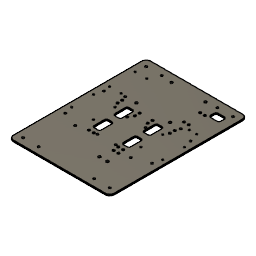
layer2_plate_v0_1 (Autodesk Fusion 360 design; units mm, degrees)
part number: 2026-05-30-13-28-22-122
Autodesk Fusion 360 part; units mm, degrees
box "长方体基本要素1" add length 285 width 145 height 3 placed x (0, 0, 1) y (1, 0, 0) z (0, 1, 0) at (0, 0, 0)
sketch "草图2" plane through (0, 3, 0) normal (0, 1, 0) x (-1, 0, 0)
  line L0 (0, 285) -> (-145, 285)
  line L1 (-145, 285) -> (-145, 0) construction
  line L2 (-145, 0) -> (0, 0)
  line L3 (0, 0) -> (0, 285) construction
  line L4 (0, 142.5) -> (-145, 142.5) construction
  line L5 (-72.5, 0) -> (-72.5, 285) construction
  line L6 (-30.4, 10) -> (-114.6, 10)
  line L7 (-114.6, 10) -> (-114.6, 97.5)
  line L8 (-114.6, 97.5) -> (-30.4, 97.5)
  line L9 (-30.4, 97.5) -> (-30.4, 10)
  line L10 (22.3, 32.5) -> (-7.7, 32.5)
  line L11 (-7.7, 32.5) -> (-7.7, 92.5)
  line L12 (-7.7, 92.5) -> (22.3, 92.5)
  line L13 (22.3, 92.5) -> (22.3, 32.5)
  line L14 (-137.6, 57.5) -> (-159.6, 57.5)
  line L15 (-159.6, 57.5) -> (-159.6, 87.5)
  line L16 (-159.6, 87.5) -> (-137.6, 87.5)
  line L17 (-137.6, 87.5) -> (-137.6, 57.5)
  line L18 (-50.8, 122.5) -> (-94.2, 122.5)
  line L19 (-94.2, 122.5) -> (-94.2, 189.43)
  line L20 (-94.2, 189.43) -> (-50.8, 189.43)
  line L21 (-50.8, 189.43) -> (-50.8, 122.5)
  line L22 (32.3, 0) -> (-177.3, 0)
  line L23 (32.3, 285) -> (-177.3, 285)
  line L24 (32.3, 0) -> (32.3, 285)
  line L25 (-177.3, 0) -> (-177.3, 285)
  line L26 (24.3, 117.5) -> (-25.7, 117.5)
  line L27 (-25.7, 167.5) -> (24.3, 167.5)
  line L28 (24.3, 167.5) -> (24.3, 117.5)
  line L29 (24.3, 142.5) -> (-24.8585, 142.5) construction
  line L30 (-25.7, 125) -> (-33.7, 125)
  line L31 (-33.7, 125) -> (-33.7, 160)
  line L32 (-33.7, 160) -> (-25.7, 160)
  line L33 (-25.7, 117.5) -> (-25.7, 125)
  line L34 (-25.7, 160) -> (-25.7, 167.5)
  line L35 (-169.3, 167.5) -> (-169.3, 117.5)
  line L36 (-169.3, 117.5) -> (-119.3, 117.5)
  line L37 (-119.3, 167.5) -> (-169.3, 167.5)
  line L38 (-119.3, 160) -> (-119.3, 167.5)
  line L39 (-111.3, 160) -> (-119.3, 160)
  line L40 (-111.3, 125) -> (-111.3, 160)
  line L41 (-119.3, 125) -> (-111.3, 125)
  line L42 (-119.3, 117.5) -> (-119.3, 125)
  line L43 (-38.25, 107) -> (-46.25, 107)
  line L44 (-49.25, 110) -> (-49.25, 132)
  line L45 (-46.25, 135) -> (-38.25, 135)
  line L46 (-35.25, 132) -> (-35.25, 110)
  arc A0 (-38.25, 107) -> (-35.25, 110) centre (-38.25, 110) ccw
  arc A1 (-49.25, 110) -> (-46.25, 107) centre (-46.25, 110) ccw
  arc A2 (-46.25, 135) -> (-49.25, 132) centre (-46.25, 132) ccw
  arc A3 (-35.25, 132) -> (-38.25, 135) centre (-38.25, 132) ccw
  line L47 (-33.7, 125) -> (-35.25, 125) construction
  line L48 (-50.8, 122.5) -> (-49.25, 122.5) construction
  line L49 (-35.25, 153) -> (-35.25, 175)
  arc A4 (-35.25, 175) -> (-38.25, 178) centre (-38.25, 175) ccw
  line L50 (-38.25, 178) -> (-46.25, 178)
  arc A5 (-46.25, 178) -> (-49.25, 175) centre (-46.25, 175) ccw
  line L51 (-49.25, 175) -> (-49.25, 153)
  arc A6 (-49.25, 153) -> (-46.25, 150) centre (-46.25, 153) ccw
  line L52 (-46.25, 150) -> (-38.25, 150)
  arc A7 (-38.25, 150) -> (-35.25, 153) centre (-38.25, 153) ccw
  line L53 (-106.75, 178) -> (-98.75, 178)
  line L54 (-106.75, 107) -> (-98.75, 107)
  arc A8 (-95.75, 132) -> (-98.75, 135) centre (-98.75, 132) ccw
  arc A9 (-98.75, 107) -> (-95.75, 110) centre (-98.75, 110) ccw
  arc A10 (-98.75, 150) -> (-95.75, 153) centre (-98.75, 153) ccw
  line L55 (-98.75, 150) -> (-106.75, 150)
  arc A11 (-109.75, 153) -> (-106.75, 150) centre (-106.75, 153) ccw
  line L56 (-109.75, 132) -> (-109.75, 110)
  arc A12 (-106.75, 135) -> (-109.75, 132) centre (-106.75, 132) ccw
  arc A13 (-95.75, 175) -> (-98.75, 178) centre (-98.75, 175) ccw
  line L57 (-98.75, 135) -> (-106.75, 135)
  arc A14 (-106.75, 178) -> (-109.75, 175) centre (-106.75, 175) ccw
  arc A15 (-109.75, 110) -> (-106.75, 107) centre (-106.75, 110) ccw
  line L58 (-95.75, 110) -> (-95.75, 132)
  line L59 (-95.75, 175) -> (-95.75, 153)
  line L60 (-109.75, 153) -> (-109.75, 175)
  line L61 (-92.5, 213.47) -> (-116.12, 213.47)
  line L62 (-116.12, 213.47) -> (-116.12, 245)
  line L63 (-116.12, 245) -> (-92.5, 245)
  line L64 (-92.5, 245) -> (-92.5, 213.47)
  line L65 (-140.3, 25) -> (-154.3, 25)
  line L66 (-157.3, 28) -> (-157.3, 36)
  line L67 (-154.3, 39) -> (-140.3, 39)
  line L68 (-137.3, 36) -> (-137.3, 28)
  circle A16 centre (-130, 15) radius 2.15
  circle A17 centre (-15, 15) radius 2.15
  circle A18 centre (-130, 270) radius 2.15
  circle A19 centre (-15, 270) radius 2.15
  arc A20 (-140.3, 25) -> (-137.3, 28) centre (-140.3, 28) ccw
  arc A21 (-137.3, 36) -> (-140.3, 39) centre (-140.3, 36) ccw
  arc A22 (-154.3, 39) -> (-157.3, 36) centre (-154.3, 36) ccw
  arc A23 (-157.3, 28) -> (-154.3, 25) centre (-154.3, 28) ccw
  circle A24 centre (-15, 90.825) radius 2.15
  circle A25 centre (-130, 90.825) radius 2.15
  circle A26 centre (-15, 194.175) radius 2.15
  circle A27 centre (-130, 194.175) radius 2.15
  circle A28 centre (17.3, 270) radius 2.15
  circle A29 centre (-162.3, 270) radius 2.15
  circle A30 centre (17.3, 15) radius 2.15
  circle A31 centre (-162.3, 15) radius 2.15
  circle A32 centre (17.3, 102.5) radius 2.15
  circle A33 centre (-162.3, 102.5) radius 2.15
  circle A34 centre (17.3, 182.5) radius 2.15
  circle A35 centre (-162.3, 182.5) radius 2.15
  circle A36 centre (19.3, 36) radius 1.75
  line L69 (22.3, 62.5) -> (-7.7, 62.5) construction
  line L70 (7.3, 32.5) -> (7.3, 92.5) construction
  circle A37 centre (-4.7, 36) radius 1.75
  circle A38 centre (19.3, 89) radius 1.75
  circle A39 centre (-4.7, 89) radius 1.75
  circle A40 centre (-141.1, 84) radius 1.65
  line L71 (-148.6, 57.5) -> (-148.6, 87.5) construction
  circle A41 centre (-156.1, 84) radius 1.65
  circle A42 centre (-96, 225.17) radius 2.65
  line L72 (-104.31, 213.47) -> (-104.31, 245) construction
  circle A43 centre (-112.62, 225.17) radius 2.65
  line L73 (-30.4, 53.75) -> (-114.6, 53.75) construction
  circle A44 centre (-37.6, 90.3) radius 2.5
  circle A45 centre (-107.4, 90.3) radius 2.5
  circle A46 centre (-37.6, 17.2) radius 2.5
  circle A47 centre (-107.4, 17.2) radius 2.5
  circle A48 centre (21.8, 120) radius 1.75
  line L74 (-0.7, 117.5) -> (-0.7, 167.5) construction
  line L75 (-0.7, 167.5) -> (-0.7, 117.5) construction
  circle A49 centre (21.8, 165) radius 1.75
  circle A50 centre (-23.2, 120) radius 1.75
  circle A51 centre (-23.2, 165) radius 1.75
  circle A52 centre (-166.8, 120) radius 1.75
  circle A53 centre (-121.8, 120) radius 1.75
  circle A54 centre (-166.8, 165) radius 1.75
  circle A55 centre (-121.8, 165) radius 1.75
  line L76 (-50.8, 155.965) -> (-94.2, 155.965) construction
  circle A56 centre (-53.6, 186.765) radius 2.15
  circle A57 centre (-91.4, 186.765) radius 2.15
  circle A58 centre (-53.6, 125.165) radius 2.15
  circle A59 centre (-91.4, 125.165) radius 2.15
  circle A60 centre (-131.1, 75.2117) radius 1.75
  circle A61 centre (-121.1, 75.2117) radius 1.75
  line L77 (-42.25, 150) -> (-42.25, 178) construction
  circle A62 centre (-37.25, 188) radius 1.75
  circle A63 centre (-107.75, 188) radius 1.75
  line L78 (-54.79, 110) -> (-91.4013, 110) construction
  circle A64 centre (-59.25, 105) radius 1.75
  circle A65 centre (-85.75, 105) radius 1.75
  circle A66 centre (-18.036, 100) radius 1.75
  line L79 (-114.6, 61.3197) -> (-137.6, 61.3197) construction
  line L80 (-126.1, 61.3197) -> (-126.1, 45.2779) construction
  circle A67 centre (-131.1, 41.8248) radius 1.75
  circle A68 centre (-121.1, 41.8248) radius 1.75
  circle A69 centre (-59.25, 115) radius 1.75
  circle A70 centre (-85.75, 115) radius 1.75
  circle A71 centre (-18.286, 110) radius 1.75
  circle A72 centre (-126.964, 100) radius 1.75
  circle A73 centre (-126.714, 110) radius 1.75
  circle A74 centre (-99.31, 199.046) radius 1.75
  circle A75 centre (-109.31, 199.046) radius 1.75
  circle A76 centre (-47.25, 188) radius 1.75
  circle A77 centre (-97.75, 188) radius 1.75
  point P0 (-109.75, 125)
  point P1 (-95.75, 122.5)
  point P2 (-137.3, 25)
  point P3 (-157.3, 25)
  point P4 (-137.3, 39)
  point P5 (-121.1, 75.2117)
  point P6 (-131.1, 75.2117)
  point P7 (-72.5, 97.5)
  point P8 (-72.5, 122.5)
  point P9 (-18.036, 100)
  point P10 (-131.1, 41.8248)
  point P11 (-121.1, 41.8248)
  dimension "d12" = 43.4
  dimension "d13" = 66.93
  dimension "d16" = 84.2
  dimension "d17" = 87.5
  dimension "d20" = 10
  dimension "d21" = 30
  dimension "d22" = 60
  dimension "d23" = 209.6
  dimension "d24" = 50
  dimension "d25" = 50
  dimension "d26" = 8
  dimension "d27" = 35
  dimension "d31" = 14
  dimension "d32" = 3
  dimension "d35" = 28
  dimension "d36" = 15
  dimension "d37" = 8
  dimension "d38" = 25
  dimension "d39" = 10
  dimension "d40" = 22
  dimension "d41" = 30
  dimension "d42" = 30
  dimension "d43" = 23
  dimension "d46" = 23.62
  dimension "d47" = 31.53
  dimension "d48" = 20
  dimension "d49" = 40
  dimension "d70" = 20
  dimension "d71" = 14
  dimension "d72" = 25
  dimension "d73" = 20
  dimension "d74" = 4.3
  dimension "d75" = 15
  dimension "d76" = 15
  dimension "d77" = 3
  dimension "d78" = 3
  dimension "d79" = 3
  dimension "d80" = 3
  dimension "d89" = 4.3
  dimension "d90" = 90.825
  dimension "d91" = 15
  dimension "d96" = 4.3
  dimension "d97" = 15
  dimension "d98" = 15
  dimension "d99" = 4.3
  dimension "d100" = 15
  dimension "d101" = 10
  dimension "d104" = 3.5
  dimension "d105" = 53
  dimension "d106" = 24
  dimension "d107" = 3.3
  dimension "d108" = 15
  dimension "d109" = 3.5
  dimension "d110" = 5.3
  dimension "d111" = 3.5
  dimension "d112" = 11.7
  dimension "d113" = 5
  dimension "d114" = 73.1
  dimension "d115" = 69.8
  dimension "d116" = 3.5
  dimension "d117" = 45
  dimension "d118" = 45
  dimension "d119" = 4.3
  dimension "d120" = 37.8
  dimension "d121" = 61.6
  dimension "d122" = 25
  dimension "d127" = 3.5
  dimension "d128" = 3.5
  dimension "d129" = 3.5
  dimension "d130" = 10
  dimension "d131" = 3.5
  dimension "d132" = 10
  dimension "d134" = 3.5
  dimension "d135" = 10
  dimension "d136" = 3.5
  dimension "d137" = 3.5
  dimension "d138" = 10
  dimension "d139" = 10
  dimension "d140" = 3.5
  dimension "d141" = 10
  dimension "d142" = 7.5
  dimension "d143" = 3.5
  dimension "d144" = 10
  dimension "d145" = 10
  constraint midpoint L3 L4.start
  constraint midpoint L1 L4.end
  constraint midpoint L2 L5.start
  constraint midpoint L0 L5.end
  constraint horizontal L6
  constraint vertical L7
  constraint horizontal L8
  constraint vertical L9
  constraint horizontal L10
  constraint vertical L11
  constraint horizontal L12
  constraint vertical L13
  constraint horizontal L14
  constraint vertical L15
  constraint horizontal L16
  constraint vertical L17
  constraint horizontal L18
  constraint vertical L19
  constraint horizontal L20
  constraint vertical L21
  constraint symmetric L5 L7 L9
  constraint parallel L6 L22
  constraint symmetric L5 L22.start L22.end
  constraint coincident L5.start L22
  constraint symmetric L4 L22.start L23.start
  constraint symmetric L4 L22.end L23.end
  constraint horizontal L26
  constraint vertical L33
  constraint horizontal L27
  constraint vertical L28
  constraint midpoint L28 L29.start
  constraint perpendicular L30 L33
  constraint perpendicular L4 L31
  constraint perpendicular L32 L34
  constraint symmetric L29 L30 L32
  constraint symmetric L4 L26 L27
  constraint collinear L33 L34
  constraint symmetric L5 L26.start L35.end
  constraint symmetric L5 L26.end L36.end
  constraint symmetric L5 L27.start L37.start
  constraint symmetric L5 L27.end L35.start
  constraint symmetric L5 L30.start L41.start
  constraint symmetric L5 L30.end L40.start
  constraint symmetric L5 L31.end L39.start
  constraint symmetric L5 L32.end L38.start
  constraint horizontal L43
  constraint vertical L44
  constraint horizontal L45
  constraint vertical L46
  constraint tangent L46 A0
  constraint tangent L43 A0
  constraint tangent L43 A1
  constraint tangent L44 A1
  constraint tangent L44 A2
  constraint tangent L45 A2
  constraint tangent L45 A3
  constraint tangent L46 A3
  constraint coincident L46 L47.end
  constraint perpendicular L46 L47
  constraint coincident L44 L48.end
  constraint perpendicular L44 L48
  constraint equal L47 L48
  constraint symmetric L5 L19 L21
  constraint symmetric L4 L46.end L49.end
  constraint symmetric L4 L43.start A4.end
  constraint symmetric L4 A0 A4
  constraint symmetric L4 L43.end L50.end
  constraint symmetric L4 L44.start A5.end
  constraint symmetric L4 A1 A5
  constraint symmetric L4 L44.end L51.end
  constraint symmetric L4 L45.start A6.end
  constraint symmetric L4 A2 A6
  constraint symmetric L4 L45.end L52.end
  constraint symmetric L4 L46.start L49.start
  constraint symmetric L4 A3 A7
  constraint symmetric L5 L46.end L56.end
  constraint symmetric L5 L43.start L54.start
  constraint symmetric L5 A0 A15
  constraint symmetric L5 L43.end L54.end
  constraint symmetric L5 L44.start A9.end
  constraint symmetric L5 A1 A9
  constraint symmetric L5 L44.end A8.start
  constraint symmetric L5 L45.start A8.end
  constraint symmetric L5 A2 A8
  constraint symmetric L5 L45.end A12.start
  constraint symmetric L5 L46.start L56.start
  constraint symmetric L5 A3 A12
  constraint symmetric L5 L47.end P0
  constraint symmetric L5 L48.end P1
  constraint symmetric L5 L49.start A11.start
  constraint symmetric L5 L49.end A14.end
  constraint symmetric L5 A4.end L53.start
  constraint symmetric L5 A4 A14
  constraint symmetric L5 L50.end L53.end
  constraint symmetric L5 A5.end A13.start
  constraint symmetric L5 A5 A13
  constraint symmetric L5 L51.end A10.end
  constraint symmetric L5 A6.end A10.start
  constraint symmetric L5 A6 A10
  constraint symmetric L5 L52.end L55.end
  constraint symmetric L5 A7 A11
  constraint equal A0 A1
  constraint equal A1 A3
  constraint equal A1 A2
  constraint horizontal L61
  constraint vertical L62
  constraint horizontal L63
  constraint vertical L64
  constraint horizontal L65
  constraint vertical L66
  constraint horizontal L67
  constraint vertical L68
  constraint symmetric L5 A16 A17
  constraint symmetric L4 A16 A18
  constraint symmetric L4 A17 A19
  constraint coincident P2 L68
  constraint coincident P2 L65
  constraint tangent L68 A20
  constraint tangent L65 A20
  constraint coincident P4 L67
  constraint coincident P4 L68
  constraint tangent L67 A21
  constraint tangent L68 A21
  constraint tangent L67 A22
  constraint tangent L66 A22
  constraint coincident P3 L65
  constraint coincident P3 L66
  constraint tangent L65 A23
  constraint tangent L66 A23
  constraint symmetric L5 A24 A25
  constraint symmetric L4 A24 A26
  constraint symmetric L4 A25 A27
  constraint symmetric L5 A28 A29
  constraint symmetric L4 A28 A30
  constraint symmetric L4 A29 A31
  constraint symmetric L5 A32 A33
  constraint symmetric L4 A32 A34
  constraint symmetric L4 A33 A35
  constraint midpoint L13 L69.start
  constraint midpoint L11 L69.end
  constraint midpoint L10 L70.start
  constraint midpoint L12 L70.end
  constraint symmetric A36 L70 A37
  constraint symmetric A36 L69 A38
  constraint symmetric L69 A37 A39
  constraint midpoint L14 L71.start
  constraint midpoint L16 L71.end
  constraint symmetric A40 L71 A41
  constraint midpoint L61 L72.start
  constraint midpoint L63 L72.end
  constraint symmetric A42 L72 A43
  constraint midpoint L9 L73.start
  constraint midpoint L7 L73.end
  constraint symmetric L5 A44 A45
  constraint symmetric L73 A44 A46
  constraint symmetric L73 A45 A47
  constraint midpoint L26 L74.start
  constraint midpoint L27 L74.end
  constraint symmetric L29 A48 A49
  constraint symmetric L29 L74.start L74.end
  constraint symmetric L29 L74.end L74.start
  constraint symmetric A48 L74 A50
  constraint symmetric L74 A49 A51
  constraint symmetric L5 A48 A52
  constraint symmetric L5 A49 A54
  constraint symmetric L5 A50 A53
  constraint symmetric L5 A51 A55
  constraint midpoint L21 L76.start
  constraint midpoint L19 L76.end
  constraint symmetric L5 A56 A57
  constraint symmetric L76 A56 A58
  constraint symmetric L76 A57 A59
  constraint coincident P6 A60.centre
  constraint coincident P5 A61.centre
  constraint midpoint L52 L77.start
  constraint midpoint L50 L77.end
  constraint symmetric L5 A62 A63
  constraint perpendicular L44 L78
  constraint midpoint L8 P7
  constraint midpoint L18 P8
  constraint symmetric L78 P7 P8
  constraint symmetric L5 A64 A65
  constraint coincident P9 A66.centre
  constraint coincident L7 L79.start
  constraint coincident L17 L79.end
  constraint perpendicular L17 L79
  constraint midpoint L79 L80.start
  constraint perpendicular L79 L80
  constraint symmetric P6 P5 L80
  constraint coincident P10 A67.centre
  constraint coincident P11 A68.centre
  constraint symmetric L80 P11 P10
  constraint symmetric L78 A64 A69
  constraint symmetric L78 A65 A70
  constraint symmetric L5 A66 A72
  constraint symmetric L5 A71 A73
  constraint symmetric L72 A74 A75
  constraint symmetric L77 A62 A76
  constraint symmetric L5 A76 A77
  measures "d12" distance of L19.end L20.end
  measures "d13" distance of L18.end L19.end
  measures "d16" distance of L7.end L8.end
  measures "d17" distance of L6.end L7.end
  measures "d20" distance of L2 L6
  measures "d21" distance of L11.end L12.end
  measures "d22" distance of L10.start L12.end
  measures "d23" distance of L22.start L22.end
  measures "d24" distance of L26.start L26.end
  measures "d25" distance of L26.start L27.end
  measures "d26" distance of L30.start L30.end
  measures "d27" distance of L30.end L31.end
  measures "d31" distance of L44 L46
  measures "d32" radius of A1
  measures "d35" distance of L43 L45
  measures "d36" distance of L45 L52
  measures "d37" distance of L24 L28
  measures "d38" distance of L12 L26
  measures "d39" distance of L13 L24
  measures "d40" distance of L14.start L14.end
  measures "d41" distance of L14.end L15.end
  measures "d42" distance of L16 L36
  measures "d43" distance of L7 L17
  measures "d46" distance of L62.end L63.end
  measures "d47" distance of L61.start L63.end
  measures "d48" distance of L5 L64
  measures "d49" distance of L23 L63
  measures "d70" distance of P2 P3
  measures "d71" distance of P2 P4
  measures "d72" distance of L22 P2
  measures "d73" distance of L25 L66
  measures "d74" diameter of A16
  measures "d75" distance of L22 A16.centre
  measures "d76" distance of L1 A16.centre
  measures "d77" radius of A20
  measures "d78" radius of A21
  measures "d79" radius of A22
  measures "d80" radius of A23
  measures "d89" diameter of A24
  measures "d90" distance of L22 A24.centre
  measures "d91" distance of L3 A24.centre
  measures "d96" diameter of A28
  measures "d97" distance of L24 A28.centre
  measures "d98" distance of L23 A28.centre
  measures "d99" diameter of A32
  measures "d100" distance of L24 A32.centre
  measures "d101" distance of L12 A32.centre
  measures "d104" diameter of A36
  measures "d105" distance of A36.centre A38.centre
  measures "d106" distance of A36.centre A37.centre
  measures "d107" diameter of A40
  measures "d108" distance of A40.centre A41.centre
  measures "d109" distance of L16 A40.centre
  measures "d110" diameter of A42
  measures "d111" distance of L64 A42.centre
  measures "d112" distance of L61 A42.centre
  measures "d113" diameter of A44
  measures "d114" distance of A44.centre A46.centre
  measures "d115" distance of A46.centre A47.centre
  measures "d116" diameter of A48
  measures "d117" distance of A48.centre A50.centre
  measures "d118" distance of A48.centre A49.centre
  measures "d119" diameter of A56
  measures "d120" distance of A56.centre A57.centre
  measures "d121" distance of A56.centre A58.centre
  measures "d122" distance of L8 L18
  measures "d127" diameter of A60
  measures "d128" diameter of A61
  measures "d129" diameter of A62
  measures "d130" distance of L50 A62.centre
  measures "d131" diameter of A64
  measures "d132" distance of L44 A64.centre
  measures "d134" diameter of A66
  measures "d135" distance of P5 P6
  measures "d136" diameter of A67
  measures "d137" diameter of A68
  measures "d138" distance of P10 P11
  measures "d139" distance of A64.centre A69.centre
  measures "d140" diameter of A71
  measures "d141" vertical distance of P9 A71.centre
  measures "d142" distance of L12 P9
  measures "d143" diameter of A74
  measures "d144" distance of A74.centre A75.centre
  measures "d145" distance of A62.centre A76.centre
extrude "拉伸3" add sketch "草图2" against normal blind 3 contours L0 L2 L22 L23 L24 L25 | L6 L7 L8 L9 | L10 L11 L12 L13 | L14 L15 L16 L17 | L18 L19 L20 L21 | L26 L27 L28 L30 L31 L32 L33 L34 | L35 L36 L37 L38 L39 L40 L41 L42 | L43 L44 L45 L46 A0 A1 A2 A3 | L49 A4 L50 A5 L51 A6 L52 A7 | L53 A10 L55 A11 A13 A14 L59 L60 | L54 A8 A9 L56 A12 L57 A15 L58 | L61 L62 L63 L64 | L65 L66 L67 L68 A20 A21 A22 A23 | A16 | A17 | A18 | A19 | A24 | A25 | A26 | A27 | A28 | A29 | A30 | A31 | A32 | A33 | A34 | A35 | A36 | A37 | A38 | A39 | A40 | A41 | A42 | A43 | A44 | A45 | A46 | A47 | A48 | A49 | A50 | A51 | A52 | A53 | A54 | A55 | A56 | A57 | A58 | A59 | A60 | A61 | A62 | A63 | A64 | A65 | A66 | A67 | A68 | A69 | A70 | A71 | A72 | A73 | A74 | A75 | A76 | A77
extrude "拉伸4" cut sketch "草图2" against normal blind 4 contours L43 L44 L45 L46 A0 A1 A2 A3 | L49 A4 L50 A5 L51 A6 L52 A7 | L53 A10 L55 A11 A13 A14 L59 L60 | L54 A8 A9 L56 A12 L57 A15 L58
fillet "圆角1" radius 10 4 edges at (177.3, 1.5, 285) (177.3, 1.5, 0) (-32.3, 1.5, 285) (-32.3, 1.5, 0)
fillet "圆角2" radius 0.5 16 edges at (49.25, 3, 121) (48.3713, 3, 134.1213) (42.25, 3, 135) (36.1287, 3, 134.1213) (35.25, 3, 121) (36.1287, 3, 107.8787) (42.25, 3, 107) (48.3713, 3, 107.8787) (35.25, 0, 121) (36.1287, 0, 134.1213) (42.25, 0, 135) (48.3713, 0, 134.1213) (49.25, 0, 121) (48.3713, 0, 107.8787) (42.25, 0, 107) (36.1287, 0, 107.8787)
fillet "圆角3" radius 0.5 16 edges at (35.25, 3, 164) (36.1287, 3, 150.8787) (42.25, 3, 150) (48.3713, 3, 150.8787) (49.25, 3, 164) (48.3713, 3, 177.1213) (42.25, 3, 178) (36.1287, 3, 177.1213) (48.3713, 0, 150.8787) (42.25, 0, 150) (36.1287, 0, 150.8787) (35.25, 0, 164) (36.1287, 0, 177.1213) (42.25, 0, 178) (48.3713, 0, 177.1213) (49.25, 0, 164)
fillet "圆角4" radius 0.5 16 edges at (102.75, 0, 178) (108.8713, 0, 177.1213) (109.75, 0, 164) (108.8713, 0, 150.8787) (102.75, 0, 150) (96.6287, 0, 150.8787) (95.75, 0, 164) (96.6287, 0, 177.1213) (96.6287, 3, 150.8787) (102.75, 3, 150) (108.8713, 3, 150.8787) (109.75, 3, 164) (108.8713, 3, 177.1213) (102.75, 3, 178) (96.6287, 3, 177.1213) (95.75, 3, 164)
fillet "圆角5" radius 0.5 16 edges at (108.8713, 3, 107.8787) (109.75, 3, 121) (108.8713, 3, 134.1213) (102.75, 3, 135) (96.6287, 3, 134.1213) (95.75, 3, 121) (96.6287, 3, 107.8787) (102.75, 3, 107) (96.6287, 0, 107.8787) (95.75, 0, 121) (96.6287, 0, 134.1213) (102.75, 0, 135) (108.8713, 0, 134.1213) (109.75, 0, 121) (108.8713, 0, 107.8787) (102.75, 0, 107)
fillet "圆角6" radius 0.5 16 edges at (-32.3, 3, 142.5) (-29.3711, 3, 2.9289) (72.5, 3, 0) (174.3711, 3, 2.9289) (177.3, 3, 142.5) (174.3711, 3, 282.0711) (72.5, 3, 285) (-29.3711, 3, 282.0711) (72.5, 0, 285) (174.3711, 0, 282.0711) (177.3, 0, 142.5) (174.3711, 0, 2.9289) (72.5, 0, 0) (-29.3711, 0, 2.9289) (-32.3, 0, 142.5) (-29.3711, 0, 282.0711)
extrude "拉伸5" cut sketch "草图2" against normal blind 3 contours L65 L66 L67 L68 A20 A21 A22 A23 | A16 | A17 | A18 | A19
fillet "圆角8" radius 0.5 16 edges at (137.3, 0, 32) (138.1787, 0, 38.1213) (147.3, 0, 39) (156.4213, 0, 38.1213) (157.3, 0, 32) (156.4213, 0, 25.8787) (147.3, 0, 25) (138.1787, 0, 25.8787) (147.3, 3, 39) (138.1787, 3, 38.1213) (137.3, 3, 32) (138.1787, 3, 25.8787) (147.3, 3, 25) (156.4213, 3, 25.8787) (157.3, 3, 32) (156.4213, 3, 38.1213)
extrude "拉伸6" cut sketch "草图2" against normal blind 3 contours A24 | A25 | A26 | A27
extrude "拉伸7" cut sketch "草图2" against normal blind 3 contours A28 | A29 | A30 | A31 | A32 | A33 | A34 | A35
extrude "拉伸8" cut sketch "草图2" against normal blind 3 contours A36 | A37 | A38 | A39 | A40 | A41 | A42 | A43 | A44 | A45 | A46 | A47 | A48 | A49 | A50 | A51 | A52 | A53 | A54 | A55 | A56 | A57 | A58 | A59
extrude "拉伸9" cut sketch "草图2" against normal blind 3 contours A60 | A61 | A62 | A63 | A64 | A65 | A66 | A67 | A68 | A69 | A70 | A71 | A72 | A73 | A74 | A75 | A76 | A77
fillet "圆角9" radius 0.5 36 edges at (38.8816, 3, 188.6328) (38.8816, 0, 187.3672) (48.8816, 0, 187.3672) (48.8816, 3, 188.6328) (99.3816, 3, 188.6328) (99.3816, 0, 187.3672) (109.3816, 0, 187.3672) (109.3816, 3, 188.6328) (100.9416, 3, 199.6788) (100.9416, 0, 198.4132) (110.9416, 3, 199.6788) (110.9416, 0, 198.4132) (60.8816, 0, 114.3672) (60.8816, 0, 104.3672) (60.8816, 3, 105.6328) (60.8816, 3, 115.6328) (87.3816, 3, 115.6328) (87.3816, 3, 105.6328) (87.3816, 0, 104.3672) (87.3816, 0, 114.3672) (19.6676, 0, 99.3672) (19.6676, 3, 100.6328) (19.9176, 0, 109.3672) (19.9176, 3, 110.6328) (122.7316, 0, 74.5789) (122.7316, 3, 75.8446) (132.7316, 0, 74.5789) (132.7316, 3, 75.8446) (122.7316, 3, 42.4576) (122.7316, 0, 41.192) (132.7316, 0, 41.192) (132.7316, 3, 42.4576) (128.3456, 0, 109.3672) (128.3456, 3, 110.6328) (128.5955, 0, 99.3672) (128.5955, 3, 100.6328)
